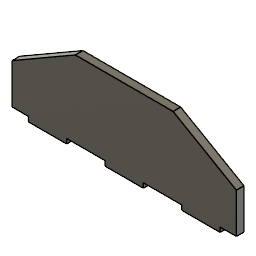
Laterales carga (Autodesk Fusion 360 design; units mm, degrees)
Autodesk Fusion 360 part; units mm, degrees
sketch "Boceto1" plane through (0, 0, 0) normal (0, 0, 1) x (1, 0, 0)
  line L0 (-58.5, 20) -> (58.5, 20)
  line L1 (58.5, 20) -> (58.5, -20)
  line L2 (58.5, -20) -> (-58.5, -20)
  line L3 (-58.5, -20) -> (-58.5, 20)
  line L4 (-58.5, 20) -> (58.5, -20) construction
  line L5 (58.5, 20) -> (-58.5, -20) construction
  dimension "d1" = 117
  dimension "d2" = 40
  constraint horizontal L0
  constraint perpendicular L0 L1
  constraint parallel L0 L2
  constraint parallel L1 L3
  constraint coincident L4 origin
  constraint coincident L5 origin
  measures "d1" distance of L1.end L2.end
  measures "d2" distance of L0.end L1.end
extrude "Extruir1" add sketch "Boceto1" along normal blind 4
sketch "Boceto2" plane through (0, 0, 4) normal (0, 0, 1) x (1, 0, 0)
  line L0 (-58.5, -20) -> (58.5, -20)
  line L1 (58.5, -20) -> (58.5, 20)
  line L2 (58.5, 20) -> (-58.5, 20)
  line L3 (-58.5, 20) -> (-58.5, -20)
  line L4 (-50, -20) -> (-30, -20)
  line L5 (-30, -20) -> (-30, -22.48)
  line L6 (-30, -22.48) -> (-50, -22.48)
  line L7 (-50, -22.48) -> (-50, -20)
  line L8 (-10, -20) -> (10, -20)
  line L9 (10, -20) -> (10, -22.48)
  line L10 (10, -22.48) -> (-10, -22.48)
  line L11 (-10, -22.48) -> (-10, -20)
  line L12 (30, -20) -> (50, -20)
  line L13 (50, -20) -> (50, -22.4109)
  line L14 (50, -22.4109) -> (30, -22.4109)
  line L15 (30, -22.4109) -> (30, -20)
  dimension "d5" = 8.5
  dimension "d6" = 20
  dimension "d7" = 20
  dimension "d8" = 20
  dimension "d9" = 20
  dimension "d10" = 20
  dimension "d11" = 8.5
  constraint horizontal L4
  constraint vertical L5
  constraint horizontal L6
  constraint vertical L7
  constraint coincident L0 L4.start
  constraint horizontal L8
  constraint vertical L9
  constraint horizontal L10
  constraint vertical L11
  constraint coincident L0 L8.start
  constraint horizontal L12
  constraint vertical L13
  constraint horizontal L14
  constraint vertical L15
  constraint coincident L0 L12.start
  measures "d5" distance of L0.start L7
  measures "d6" distance of L5.end L6.end
  measures "d7" distance of L5 L11
  measures "d8" distance of L9.end L10.end
  measures "d9" distance of L13.end L14.end
  measures "d10" distance of L9 L15
  measures "d11" distance of L0.end L13
extrude "Extruir2" add sketch "Boceto2" against normal blind 4 contours L0 L4 L5 L6 L7 | L0 L8 L9 L10 L11 | L0 L12 L13 L14 L15
sketch "Boceto3" plane through (0, 0, 4) normal (0, 0, 1) x (1, 0, 0)
  line L0 (-58.5, 0.9474) -> (-25.5, 20)
  line L1 (25.5, 20) -> (58.5, 0.9474)
  line L2 (-58.5, 20) -> (58.5, 20)
  line L3 (-58.5, 20) -> (-58.5, 0.9474)
  line L4 (-58.5, 20) -> (-25.5, 20)
  line L5 (58.5, 20) -> (58.5, 0.9474)
  point P0 (58.5, 20)
  dimension "d14" = 30
  dimension "d15" = 30
  dimension "d16" = 33
  dimension "d17" = 33
  constraint coincident L2.start L3.start
  constraint perpendicular L2 L3
  constraint coincident P0 L2.end
  constraint perpendicular L2 L5
  measures "d14" angle of L0 L2
  measures "d15" angle of L1 L2
  measures "d16" distance of L0.end L2.start
  measures "d17" distance of L1.start P0
extrude "Extruir3" cut sketch "Boceto3" against normal through all
